A side sample mold v1 (Autodesk Fusion 360 design; units mm, degrees)
Autodesk Fusion 360 part; units mm, degrees
sketch "Sketch1" plane through (0, 0, 0) normal (0, 0, 1) x (1, 0, 0)
  line L0 (125, -125) -> (-125, -125)
  line L1 (-125, -125) -> (-125, 125)
  line L2 (-125, 125) -> (125, 125)
  line L3 (125, 125) -> (125, -125)
  line L4 (125, -125) -> (-125, 125) construction
  line L5 (-125, -125) -> (125, 125) construction
  dimension "d1" = 250
  dimension "d2" = 250
  constraint horizontal L0
  constraint perpendicular L0 L1
  constraint parallel L0 L2
  constraint parallel L1 L3
  constraint coincident L4 origin
  constraint coincident L5 origin
  measures "d1" distance of L1.end L2.end
  measures "d2" distance of L0.end L1.end
extrude "Extrude1" add sketch "Sketch1" along normal blind 100
